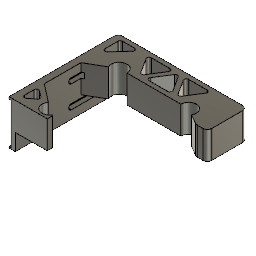
Z_Axis_SensorClipOn (Autodesk Fusion 360 design; units mm, degrees)
Autodesk Fusion 360 part; units mm, degrees
sketch "Sketch1" plane through (0, 0, 0) normal (0, 0, 1) x (1, 0, 0)
  line L0 (69.2401, 97.5535) -> (12.2401, 97.5535)
  line L1 (12.2401, 97.5535) -> (12.2401, 48.4535)
  line L2 (52.8401, 84.1535) -> (28.6401, 84.1535)
  line L3 (59.3712, 82.4035) -> (64.1343, 79.6535)
  line L4 (64.1343, 79.6535) -> (69.2401, 79.6535)
  line L5 (69.2401, 79.6535) -> (69.2401, 97.5535)
  line L6 (22.109, 82.4035) -> (14.2401, 77.8603)
  line L7 (14.2401, 77.8603) -> (14.2401, 61.3991)
  line L8 (14.2401, 61.3991) -> (22.3734, 55.0972)
  line L9 (28.5401, 52.1228) -> (28.5401, 48.4535)
  line L10 (28.5401, 48.4535) -> (12.2401, 48.4535)
  arc A0 (59.3712, 82.4035) -> (52.8401, 84.1535) centre (56.3401, 84.1535) ccw
  arc A1 (28.6401, 84.1535) -> (22.109, 82.4035) centre (25.1401, 84.1535) ccw
  arc A2 (22.3734, 55.0972) -> (28.5401, 52.1228) centre (25.1401, 52.9535) ccw
  line L11 (14.2401, 50.4535) -> (14.2401, 58.869)
  line L12 (14.2401, 58.869) -> (19.6401, 54.6849)
  line L13 (19.6401, 54.6849) -> (14.2401, 50.4535)
  line L14 (14.2401, 86.1535) -> (22.9682, 95.5535)
  line L15 (22.9682, 95.5535) -> (14.2401, 95.5535)
  line L16 (14.2401, 95.5535) -> (14.2401, 86.1535)
  line L17 (26.3674, 95.5535) -> (32.3674, 86.1535)
  line L18 (32.3674, 86.1535) -> (38.3674, 95.5535)
  line L19 (38.3674, 95.5535) -> (26.3674, 95.5535)
  line L20 (49.1128, 86.1535) -> (55.1128, 95.5535)
  line L21 (55.1128, 95.5535) -> (43.1128, 95.5535)
  line L22 (43.1128, 95.5535) -> (49.1128, 86.1535)
  line L23 (34.7401, 86.1535) -> (46.7401, 86.1535)
  line L24 (46.7401, 86.1535) -> (40.7401, 95.5535)
  line L25 (40.7401, 95.5535) -> (34.7401, 86.1535)
  dimension "d1" = 7
  dimension "d2" = 7
  dimension "d3" = 31.2
  dimension "d10" = 7
  dimension "d11" = 150
  dimension "d12" = 150
  dimension "d13" = 127.769
  dimension "d14" = 12.9
  dimension "d15" = 12.9
  dimension "d16" = 31.2
  dimension "d17" = 4.5
  dimension "d18" = 13.4
  dimension "d19" = 12.9
  dimension "d21" = 4.5
  dimension "d23" = 2
  dimension "d24" = 5.5
  dimension "d25" = 2
  dimension "d26" = 2
  dimension "d27" = 2
  dimension "d35" = 2
  dimension "d36" = 2
  dimension "d37" = 2
  dimension "d38" = 2
  dimension "d39" = 2
  dimension "d40" = 2
  dimension "d41" = 2
  dimension "d42" = 2
  dimension "d43" = 2
  dimension "d44" = 2
  dimension "d45" = 12
  dimension "d46" = 15.6
  dimension "d47" = 2
  dimension "d74" = 90
  dimension "d77" = 3.4
  constraint horizontal L2
  constraint coincident A1.centre L2
  constraint coincident A0.centre L2
  constraint horizontal L4
  constraint perpendicular L4 L5
  constraint coincident A0.centre L3
  constraint parallel L1 L7
  constraint coincident A2.centre L8
  constraint coincident A1.centre L6
  constraint perpendicular L0 L1
  constraint perpendicular L0 L5
  constraint coincident L1.end L10.end
  constraint coincident L0.start L5.end
  constraint vertical L11
  constraint parallel L8 L12
  constraint horizontal L15
  constraint perpendicular L15 L16
  constraint perpendicular L16 L19
  constraint parallel L19 L21
  constraint parallel L21 L23
  constraint parallel L18 L25
  constraint parallel L22 L24
  constraint equal L24 L25
  constraint equal L20 L22
  constraint equal L17 L18
  constraint perpendicular L1 L10
  measures "d1" diameter of A1
  measures "d2" diameter of A2
  measures "d3" distance of A1.centre A2.centre
  measures "d10" diameter of A0
  measures "d11" angle of L2 L3
  measures "d12" angle of L2 L6
  measures "d14" distance of A2.centre L1
  measures "d15" distance of A1.centre L1
  measures "d16" distance of A1.centre A0.centre
  measures "d17" distance of A2.centre L10
  measures "d18" distance of L0 L2
  measures "d19" distance of A0.centre L5
  measures "d21" distance of L2 L3.end
  measures "d23" distance of L1 L7
  measures "d24" horizontal distance of A2.centre L12.end
  measures "d25" distance of L1 L11
  measures "d26" distance of L8 L12
  measures "d27" distance of L10 L11.start
  measures "d35" distance of L0 L15
  measures "d36" distance of L1 L16
  measures "d37" distance of L0 L19
  measures "d38" distance of L0 L21
  measures "d39" distance of L2 L23
  measures "d40" distance of L2 L17.end
  measures "d41" distance of L2 L20.start
  measures "d42" distance of L0 L24.end
  measures "d43" distance of L18 L25
  measures "d44" distance of L22 L24
  measures "d45" distance of L23.start L23.end
  measures "d46" horizontal distance of A1.centre L24.end
  measures "d47" distance of L2 L14.start
  measures "d74" angle of L9 L10
  measures "d77" distance of A2.centre L9
extrude "Extrude1" add sketch "Sketch1" along normal blind 12.5
sketch "Sketch2" plane through (0, 97.5535, 0) normal (0, 1, 0) x (-1, 0, 0)
  line L0 (-69.2401, 0) -> (-12.2401, 0)
  line L1 (-12.2401, 0) -> (-12.2401, 12.5)
  line L2 (-12.2401, 12.5) -> (-69.2401, 12.5)
  line L3 (-69.2401, 12.5) -> (-69.2401, 0)
  point P0 (-60.2401, 4.5)
  dimension "d30" = 9
  dimension "d31" = 8
  measures "d30" distance of L3 P0
  measures "d31" distance of L2 P0
hole "Hole1" at (60.2401, 97.5535, 4.5) direction (0, -1, 0) diameter 5 depth 10 tip angle 118
fillet "Fillet2" radius 1 15 edges at (55.1128, 95.5535, 6.25) (43.1128, 95.5535, 6.25) (49.1128, 86.1535, 6.25) (46.7401, 86.1535, 6.25) (40.7401, 95.5535, 6.25) (34.7401, 86.1535, 6.25) (38.3674, 95.5535, 6.25) (32.3674, 86.1535, 6.25) (26.3674, 95.5535, 6.25) (22.9682, 95.5535, 6.25) (14.2401, 86.1535, 6.25) (14.2401, 95.5535, 6.25) (19.6401, 54.6849, 6.25) (14.2401, 58.869, 6.25) (14.2401, 50.4535, 6.25)
sketch "Sketch3" plane through (0, 0, 0) normal (0, 0, -1) x (1, 0, 0)
  line L0 (69.2401, -79.6535) -> (64.1343, -79.6535)
  line L1 (64.1343, -79.6535) -> (59.3712, -82.4035)
  arc A0 (52.8401, -84.1535) -> (59.3712, -82.4035) centre (56.3401, -84.1535) ccw
  line L2 (52.8401, -84.1535) -> (28.6401, -84.1535)
  arc A1 (22.109, -82.4035) -> (28.6401, -84.1535) centre (25.1401, -84.1535) ccw
  line L3 (22.109, -82.4035) -> (14.2401, -77.8603)
  line L4 (14.2401, -77.8603) -> (14.2401, -61.3991)
  line L5 (14.2401, -61.3991) -> (22.3734, -55.0972)
  arc A2 (28.5401, -52.1228) -> (22.3734, -55.0972) centre (25.1401, -52.9535) ccw
  line L6 (28.5401, -52.1228) -> (28.5401, -48.4535)
  line L7 (28.5401, -48.4535) -> (12.2401, -48.4535)
  line L8 (12.2401, -48.4535) -> (12.2401, -97.5535)
  line L9 (12.2401, -97.5535) -> (69.2401, -97.5535)
  line L10 (69.2401, -97.5535) -> (69.2401, -79.6535)
  arc A3 (27.3491, -94.0154) -> (28.1921, -95.5535) centre (28.1921, -94.5535) ccw
  line L11 (27.3491, -94.0154) -> (31.5245, -87.474)
  arc A4 (33.2103, -87.474) -> (31.5245, -87.474) centre (32.3674, -88.0121) ccw
  line L12 (33.2103, -87.474) -> (37.3857, -94.0154)
  arc A5 (36.5428, -95.5535) -> (37.3857, -94.0154) centre (36.5428, -94.5535) ccw
  line L13 (36.5428, -95.5535) -> (28.1921, -95.5535)
  arc A6 (14.2401, -56.8291) -> (15.8526, -57.6196) centre (15.2401, -56.8291) ccw
  line L14 (14.2401, -56.8291) -> (14.2401, -52.5075)
  arc A7 (15.8569, -51.7204) -> (14.2401, -52.5075) centre (15.2401, -52.5075) ccw
  line L15 (15.8569, -51.7204) -> (18.6299, -53.8933)
  arc A8 (18.6256, -55.4709) -> (18.6299, -53.8933) centre (18.0131, -54.6805) ccw
  line L16 (18.6256, -55.4709) -> (15.8526, -57.6196)
  arc A9 (15.9729, -88.0197) -> (14.2401, -88.7001) centre (15.2401, -88.7001) ccw
  line L17 (15.9729, -88.0197) -> (21.4079, -93.873)
  arc A10 (20.6751, -95.5535) -> (21.4079, -93.873) centre (20.6751, -94.5535) ccw
  line L18 (20.6751, -95.5535) -> (15.2401, -95.5535)
  arc A11 (14.2401, -94.5535) -> (15.2401, -95.5535) centre (15.2401, -94.5535) ccw
  line L19 (14.2401, -94.5535) -> (14.2401, -88.7001)
  arc A12 (49.9557, -87.474) -> (48.2699, -87.474) centre (49.1128, -88.0121) ccw
  line L20 (49.9557, -87.474) -> (54.1311, -94.0154)
  arc A13 (53.2882, -95.5535) -> (54.1311, -94.0154) centre (53.2882, -94.5535) ccw
  line L21 (53.2882, -95.5535) -> (44.9375, -95.5535)
  arc A14 (44.0945, -94.0154) -> (44.9375, -95.5535) centre (44.9375, -94.5535) ccw
  line L22 (44.0945, -94.0154) -> (48.2699, -87.474)
  arc A15 (36.5648, -86.1535) -> (35.7218, -87.6915) centre (36.5648, -87.1535) ccw
  line L23 (36.5648, -86.1535) -> (44.9155, -86.1535)
  arc A16 (45.7584, -87.6915) -> (44.9155, -86.1535) centre (44.9155, -87.1535) ccw
  line L24 (45.7584, -87.6915) -> (41.583, -94.2329)
  arc A17 (39.8972, -94.2329) -> (41.583, -94.2329) centre (40.7401, -93.6948) ccw
  line L25 (39.8972, -94.2329) -> (35.7218, -87.6915)
  line L26 (12.2401, -48.4535) -> (14.2401, -48.4535)
  line L27 (12.2401, -48.4535) -> (12.2401, -97.5535)
  line L28 (12.2401, -97.5535) -> (14.2401, -97.5535)
  line L29 (14.2401, -97.5535) -> (14.2401, -48.4535)
  dimension "d51" = 2
  dimension "d52" = 2
  constraint coincident L7.end L8.start
  constraint perpendicular L8 L26
  constraint coincident L8.end L9.start
  constraint perpendicular L27 L28
  measures "d51" distance of L7.end L26.end
  measures "d52" distance of L8.end L28.end
extrude "Extrude2" add sketch "Sketch3" along normal blind 7.5 contours L4 L7 L8 L9 L14 L19 L26 L27 L28 L29
sketch "Sketch4" plane through (12.2401, 0, 0) normal (-1, 0, 0) x (0, -1, 0)
  line L0 (-48.4535, -7.5) -> (-48.4535, 12.5)
  line L1 (-48.4535, 12.5) -> (-97.5535, 12.5)
  line L2 (-97.5535, 12.5) -> (-97.5535, -7.5)
  line L3 (-97.5535, -7.5) -> (-48.4535, -7.5)
  line L4 (-93.5535, -1.3) -> (-73.5535, -1.3)
  arc A0 (-73.5535, -3.7) -> (-73.5535, -1.3) centre (-73.5535, -2.5) ccw
  line L5 (-73.5535, -3.7) -> (-93.5535, -3.7)
  arc A1 (-93.5535, -1.3) -> (-93.5535, -3.7) centre (-93.5535, -2.5) ccw
  arc A2 (-93.5535, 8.8) -> (-93.5535, 6.4) centre (-93.5535, 7.6) ccw
  arc A3 (-73.5535, 6.4) -> (-73.5535, 8.8) centre (-73.5535, 7.6) ccw
  line L6 (-73.5535, 6.4) -> (-93.5535, 6.4)
  line L7 (-93.5535, 8.8) -> (-73.5535, 8.8)
  line L8 (-97.5535, 12.5) -> (-48.4535, 12.5)
  line L9 (-48.4535, 12.5) -> (-48.4535, 11.5)
  line L10 (-48.4535, 11.5) -> (-97.5535, 11.5)
  line L11 (-97.5535, 11.5) -> (-97.5535, 12.5)
  line L12 (-97.5535, -7.5) -> (-48.4535, -7.5)
  line L13 (-48.4535, -7.5) -> (-48.4535, -6.9)
  line L14 (-48.4535, -6.9) -> (-97.5535, -6.9)
  line L15 (-97.5535, -6.9) -> (-97.5535, -7.5)
  dimension "d55" = 2.4
  dimension "d56" = 20
  dimension "d59" = 2.4
  dimension "d60" = 20
  dimension "d61" = 7.7
  dimension "d63" = 4
  dimension "d64" = 4
  dimension "d65" = 3.7
  dimension "d69" = 1
  dimension "d79" = 0.6
  constraint horizontal L4
  constraint tangent L4 A0
  constraint tangent A0 L5
  constraint parallel L4 L5
  constraint tangent L5 A1
  constraint tangent L4 A1
  constraint horizontal L7
  constraint tangent A3 L7
  constraint tangent A3 L6
  constraint parallel L6 L7
  constraint tangent A2 L6
  constraint tangent A2 L7
  constraint horizontal L8
  constraint vertical L9
  constraint horizontal L10
  constraint vertical L11
  constraint coincident L0 L9.end
  constraint coincident L1.end L2.start
  constraint horizontal L12
  constraint vertical L13
  constraint horizontal L14
  constraint vertical L15
  constraint coincident L0 L13.end
  constraint coincident L2.end L3.start
  measures "d55" distance of L4 L5
  measures "d56" distance of A0.centre A1.centre
  measures "d59" distance of L6 L7
  measures "d60" distance of A2.centre A3.centre
  measures "d61" distance of L4 L6
  measures "d63" distance of L2 A2.centre
  measures "d64" distance of L2 A1.centre
  measures "d65" distance of L1 L7
  measures "d69" distance of L8 L10
  measures "d79" distance of L12 L14
extrude "Extrude3" cut sketch "Sketch4" against normal blind 3 contours L4 A0 L5 A1 | A2 A3 L6 L7
extrude "Extrude4" add sketch "Sketch4" along normal blind 1 contours L0 L2 L3 L12 L13 L14 L15 | L0 L1 L2 L8 L9 L10 L11
fillet "Fillet3" radius 2 3 edges at (11.2401, 97.5535, -7.2) (11.2401, 97.5535, 12) (12.2401, 97.5535, 2.3)
fillet "Fillet3" radius 2 3 edges at (69.2401, 97.5535, 6.25) (69.2401, 79.6535, 6.25) (64.1343, 79.6535, 6.25)
fillet "Fillet3" radius 0.3 1 edges at (28.5401, 52.1228, 6.25)
